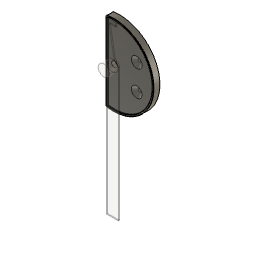
model (Autodesk Fusion 360 design; units mm, degrees)
Autodesk Fusion 360 part; units mm, degrees
sketch "Sketch1" plane through (0, 0, 0) normal (0, 1, 0) x (1, 0, 0)
  arc A0 (0, -88.9044) -> (0, 0) centre (7, -44.4522) ccw
  line L0 (0, 0) -> (0, -88.9044)
  line L1 (0, 0) -> (0, 109.0956)
  line L2 (0, 109.0956) -> (14, 109.0956)
  line L3 (14, 109.0956) -> (14, -46.4522)
  line L4 (9, -51.4522) -> (3.25, -85.2804)
  arc A1 (9, -51.4522) -> (14, -46.4522) centre (7, -44.4522) ccw
  line L5 (0, -44.4522) -> (7, -44.4522) construction
  arc A2 (3.25, -85.2804) -> (11, -85.2566) centre (7, -44.4522) ccw
  line L6 (11, -85.2566) -> (11, -89.2741)
  circle A3 centre (7, -44.4522) radius 6.6
  point P0 (52, -44.4522)
  dimension "d1" = 7
  dimension "d2" = 52
  dimension "d3" = 14
  dimension "d4" = 198
  dimension "d5" = 2
  dimension "d6" = 2
  dimension "d7" = 3.25
  dimension "d8" = 45
  dimension "d9" = 41
  dimension "d10" = 11
  dimension "d11" = 13.2
  constraint coincident A0.end L0.start
  constraint vertical L0
  constraint coincident A0.centre A1.centre
  constraint midpoint L0 L5.start
  constraint midpoint A0 P0
  constraint vertical L1
  constraint vertical L3
  constraint horizontal L2
  constraint coincident A0 L6.end
  constraint vertical L6
  measures "d1" distance of A0.centre L5.start
  measures "d2" distance of L5.start P0
  measures "d3" distance of L1.end L2.end
  measures "d4" distance of A0.start L1.end
  measures "d5" vertical distance of A0.centre L3.end
  measures "d6" horizontal distance of A0.centre L4.start
  measures "d7" distance of L0 L4.end
  measures "d8" radius of A0
  measures "d9" radius of A2
  measures "d10" horizontal distance of A0.start A2.end
  measures "d11" diameter of A3
extrude "Extrude1" add sketch "Sketch1" along normal blind 1.2 contours A0 L0 L3 L4 A1 A2 L6 | A0 L3 L4 A1 A2 L6 | A3 makes body 1
extrude "Extrude2" add sketch "Sketch1" against normal blind 1.2 separate body contours A0 L0 L3 L4 A1 A2 L6 | A0 L1 L2 L3 | A3 makes body 2
extrude "Extrude3" add sketch "Sketch1" against normal blind 10 from surface at -1.2 separate body contours A3 makes body 3
combine "Combine1" operation add target body 3 tool bodies 2 1
sketch "Sketch2" plane through (0, 1.2, 0) normal (0, 1, 0) x (-1, 0, 0)
  line L0 (0, 0) -> (0, 88.9044)
  arc A0 (0, 88.9044) -> (0, 0) centre (-7, 44.4522) ccw
  arc A1 (2, 90.5825) -> (2, -1.678) centre (-7, 44.4522) ccw
  line L1 (2, -1.678) -> (2, 90.5825)
  arc A2 (0.2, 89.0751) -> (0.2, -0.1706) centre (-7, 44.4522) ccw
  line L2 (0.2, -0.1706) -> (0.2, 89.0751)
  circle A3 centre (-7, 44.4522) radius 3.25
  circle A4 centre (-32.9808, 59.4522) radius 2.25
  circle A5 centre (-32.9808, 29.4522) radius 2.25
  line L3 (-32.9808, 29.4522) -> (-32.9808, 59.4522) construction
  line L4 (-32.9808, 59.4522) -> (-7, 44.4522) construction
  line L5 (-7, 44.4522) -> (-32.9808, 29.4522) construction
  circle A6 centre (-32.9808, 59.4522) radius 5.75 construction
  dimension "d23" = 2
  dimension "d24" = 0.2
  dimension "d25" = 6.5
  dimension "d26" = 4.5
  dimension "d27" = 11.5
  dimension "d28" = 30
  constraint concentric A0 A3
  constraint equal A4 A5
  constraint coincident A5.centre L3.start
  constraint coincident A4.centre L3.end
  constraint coincident A0.centre A1.centre
  constraint equal L4 L5
  constraint equal L3 L4
  constraint vertical L3
  constraint concentric A4 A6
  measures "d25" diameter of A3
  measures "d26" diameter of A4
  measures "d27" diameter of A6
  measures "d28" distance of A5.centre A4.centre
extrude "Extrude4" add sketch "Sketch2" along normal blind 6 separate body contours L0 A0 | A1 L1 | A2 L2 | A3 makes body 4
extrude "Extrude5" add sketch "Sketch2" against normal up to surface (1.2 mm away) contours A1 L1 bodies 4
extrude "Extrude6" cut sketch "Sketch2" along normal blind 4 contours A3 bodies 4
chamfer "Chamfer1" distance 4 angle 45 2 edges at (35.0785, 1.2, 60.2659) (35.0785, 1.2, 30.2659) on bodies 4
fillet "Fillet3" radius 2 2 edges at (-2, 3.6, 90.5825) (-2, 3.6, -1.678) on bodies 4
chamfer "Chamfer2" distance 0.25 angle 45 6 edges at (54, 0, 44.4522) (-1.5202, 0, -1.2996) (-2, 0, 44.4522) (-1.5202, 0, 90.204) (52.2, 0, 44.4522) (-0.2, 0, 44.4522) on bodies 4
equation "d1 = d3 / 2"
equation "d9 = d8 - 4 mm"
